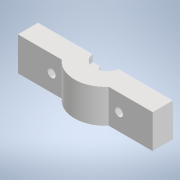
# Autodesk Inventor part: 20_Base_Sopra
Saved by Autodesk Inventor 2020.2 (Build 242310000, 310)
## iProperties
Created: 2019-10-25
Part Number: 20_Base_Sopra
Material: PLA(Stampato)(D0,646)
Document SubType Name: Modeling
Designer: socci
Density: 0.646 g/cm^3
Appearance: Default(1)
Author: socci
Autodesk Inventor part; units mm, degrees
ref_plane "YZ Plane" through (0, 0, 0) normal (1, 0, 0) x (0, 1, 0)
ref_plane "XZ Plane" through (0, 0, 0) normal (0, 1, 0) x (-1, 0, 0)
ref_plane "XY Plane" through (0, 0, 0) normal (0, 0, 1) x (1, 0, 0)
sketch "Schizzo1" plane through (0, 0, 0) normal (0, 0, 1) x (1, 0, 0)
  line L0 (50, -12.5) -> (-50, -12.5)
  line L1 (-50, -12.5) -> (-50, 12.5)
  line L2 (-50, 12.5) -> (50, 12.5)
  line L3 (50, 12.5) -> (50, -12.5)
  line L4 (50, -12.5) -> (-50, 12.5) construction
  line L5 (-50, -12.5) -> (50, 12.5) construction
  point P0 (0, 0)
  dimension "d0" = 100
  dimension "d1" = 25
  constraints: 12 end point, 2 midpoint, 2 parallel, 1 horizontal, 1 perpendicular
  measures "d0" distance of L1.end L2.end
  measures "d1" distance of L2.end L0.start
extrude "Estrusione1" add sketch "Schizzo1" along normal blind 15
sketch "Schizzo2" plane through (-50, 12.5, 0) normal (0, 1, 0) x (1, 0, 0)
  line L0 (50, 0) -> (50, 1)
  line L1 (50, 0) -> (51, 0) construction
  circle A0 centre (50, 1) radius 9.5
  dimension "d4" = 1
  dimension "d5" = 90
  dimension "d6" = 19
  constraints: 4 end point, 1 centre point, 1 coincident, 1 horizontal, 1 perpendicular, 1 vertical
  measures "d4" distance of L0.start L0.end
  measures "d5" angle of L1 L0
  measures "d6" diameter of A0
extrude "Estrusione2" cut sketch "Schizzo2" against normal blind 5
sketch "Schizzo3" plane through (-50, 7.5, 0) normal (0, 1, 0) x (1, 0, 0)
  line L0 (50, 0) -> (50, 1)
  line L1 (50, 0) -> (51, 0) construction
  circle A0 centre (50, 1) radius 4
  dimension "d9" = 1
  dimension "d10" = 90
  dimension "d11" = 8
  constraints: 4 end point, 1 centre point, 1 coincident, 1 horizontal, 1 perpendicular, 1 vertical
  measures "d9" distance of L0.start L0.end
  measures "d10" angle of L1 L0
  measures "d11" diameter of A0
extrude "Estrusione3" cut sketch "Schizzo3" against normal blind 20
sketch "Schizzo4" plane through (0, 0, 15) normal (0, 0, 1) x (1, 0, 0)
  line L0 (-25, 0) -> (25, 0)
  line L1 (-25, 0) -> (25, 0) construction
  line L2 (50, 12.5) -> (-50, 12.5) projected
  point P0 (0, 0)
  point P1 (0, 0)
  dimension "d14" = 50
  dimension "d15" = 0
  constraints: 4 end point, 2 horizontal, 1 coincident, 1 collinear, 1 midpoint, 1 parallel
  measures "d14" distance of L0.start L0.end
  measures "d15" distance between parallel lines of L0 L1
hole "Foro1" at (-25, 0, 15) at (25, 0, 15) direction (0, 0, -1) diameter 5.9 end through all clearance for "Bullone a testa esagonale" size "M5" standard "ANSI - Profilo M Metrico"
sketch "Schizzo5" plane through (-50, 12.5, 15) normal (0, 1, 0) x (1, 0, 0)
  circle A0 centre (50, 15) radius 23
  line L0 (100, 0) -> (0, 0) projected
  line L1 (67.4356, 0) -> (32.5644, 0)
  point P0 (50, 15)
  dimension "d23" = 46
  constraints: 2 end point, 2 point on circle, 2 point on line, 1 centre point, 1 coincident
  measures "d23" diameter of A0
extrude "Estrusione4" add sketch "Schizzo5" against normal blind 25 contours L0 A0 picked at (45.5796, -1.264)
